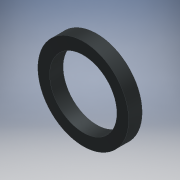
# Autodesk Inventor part: Diffbox_bear_6704DD
Saved by Autodesk Inventor 2018 (Build 220112000, 112)
## iProperties
Created: 2017-10-20
Part Number: Diffbox_bear_6704DD
Material: 鉄、ねずみ鋳鉄
Document SubType Name: Modeling
Designer: 翔
Density: 7.15 g/cm^3
Appearance: 鉄 ねずみ鋳鉄
Author: 翔
Autodesk Inventor part; units mm, degrees
ref_plane "YZ Plane" through (0, 0, 0) normal (1, 0, 0) x (0, 1, 0)
ref_plane "XZ Plane" through (0, 0, 0) normal (0, 1, 0) x (-1, 0, 0)
ref_plane "XY Plane" through (0, 0, 0) normal (0, 0, 1) x (1, 0, 0)
sketch "スケッチ1" plane through (0, 0, 0) normal (0, 0, 1) x (1, 0, 0)
  line L0 (0, 29.6124) -> (0, -32.1403)
  line L1 (10, 0) -> (10, 4)
  line L2 (10, 4) -> (13.5, 4)
  line L3 (13.5, 4) -> (13.5, 0)
  line L4 (13.5, 0) -> (10, 0)
  point P0 (0, 0)
  dimension "d0" = 10
  dimension "d1" = 4
  dimension "d2" = 13.5
  constraints: 10 end point, 3 perpendicular, 2 vertical
  measures "d0" distance between parallel lines of L0 L1
  measures "d1" distance between parallel lines of L2 L4
  measures "d2" distance between parallel lines of L3 L0
revolve "回転1" add sketch "スケッチ1" angle 360 about axis through (0, 29.6124, 0) along (0, -1, 0)
